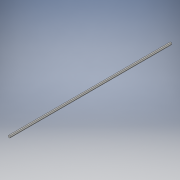
# Autodesk Inventor part: hex axle for elevator
Saved by Autodesk Inventor 2016 SP2 (Build 200236200, 236)
## iProperties
Created: 2018-01-27
Part Number: hex axle for elevator
Material: Generic
Document SubType Name: Modeling
Designer: CAD
Density: 1 g/cm^3
Appearance: Default
Author: CAD
Autodesk Inventor part; units mm, degrees
ref_plane "YZ Plane" through (0, 0, 0) normal (1, 0, 0) x (0, 1, 0)
ref_plane "XZ Plane" through (0, 0, 0) normal (0, 1, 0) x (-1, 0, 0)
ref_plane "XY Plane" through (0, 0, 0) normal (0, 0, 1) x (1, 0, 0)
sketch "Sketch1" plane through (0, 0, 0) normal (0, 0, 1) x (1, 0, 0)
  line L0 (-1.8331, 3.175) -> (1.8331, 3.175)
  line L1 (1.8331, 3.175) -> (3.6662, 0)
  line L2 (3.6662, 0) -> (1.8331, -3.175)
  line L3 (1.8331, -3.175) -> (-1.8331, -3.175)
  line L4 (-1.8331, -3.175) -> (-3.6662, 0)
  line L5 (-3.6662, 0) -> (-1.8331, 3.175)
  point P0 (0, 0)
  point P1 (0, 0)
  dimension "d0" = 6.35
  constraints: 12 end point, 1 coincident, 1 horizontal, 13 other
  measures "d0" distance between parallel lines of L3 L0
extrude "Extrusion1" add sketch "Sketch1" along normal blind 533.4
body "Solid1"
